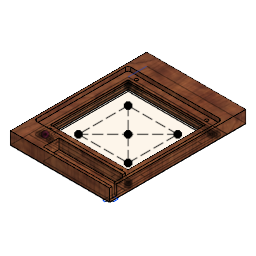
unicorn-frame-v34 (Autodesk Fusion 360 design; units mm, degrees)
Autodesk Fusion 360 part; units mm, degrees
sketch "Sketch1" plane through (0, 0, 0) normal (0, 0, 1) x (1, 0, 0)
  line L0 (0, 0) -> (254, 0)
  line L1 (254, 0) -> (254, 254)
  line L2 (254, 254) -> (0, 254)
  line L3 (0, 254) -> (0, 0)
  line L4 (279.4, 279.4) -> (-25.4, 279.4)
  line L5 (-25.4, 279.4) -> (-25.4, -25.4)
  line L6 (-25.4, -25.4) -> (279.4, -25.4)
  line L7 (279.4, -25.4) -> (279.4, 279.4)
  line L8 (246.0625, 246.0625) -> (7.9375, 246.0625)
  line L9 (7.9375, 246.0625) -> (7.9375, 7.9375)
  line L10 (7.9375, 7.9375) -> (246.0625, 7.9375)
  line L11 (246.0625, 7.9375) -> (246.0625, 246.0625)
  line L12 (258.7625, 265.1125) -> (-4.7625, 265.1125)
  line L13 (-11.1125, 258.7625) -> (-11.1125, -4.7625)
  line L14 (-4.7625, -11.1125) -> (258.7625, -11.1125)
  line L15 (265.1125, -4.7625) -> (265.1125, 258.7625)
  line L16 (39.6875, 0) -> (39.6875, -11.1125)
  line L17 (0, 39.6875) -> (-11.1125, 39.6875)
  line L18 (214.3125, 0) -> (214.3125, -11.1125)
  line L19 (254, 39.6875) -> (265.1125, 39.6875)
  line L20 (254, 214.3125) -> (265.1125, 214.3125)
  line L21 (214.3125, 254) -> (214.3125, 265.1125)
  line L22 (39.6875, 265.1125) -> (39.6875, 254)
  line L23 (-11.1125, 214.3125) -> (0, 214.3125)
  line L24 (263.525, 271.4625) -> (-9.525, 271.4625)
  line L25 (-17.4625, 263.525) -> (-17.4625, -9.525)
  line L26 (-9.525, -17.4625) -> (263.525, -17.4625)
  line L27 (271.4625, -9.525) -> (271.4625, 263.525)
  circle A0 centre (0, 0) radius 3.9688
  circle A1 centre (254, 0) radius 3.9688
  circle A2 centre (254, 254) radius 3.9688
  circle A3 centre (0, 254) radius 3.9688
  line L28 (0, 0) -> (0, -11.1125) construction
  line L29 (39.6875, -5.5563) -> (0, -5.5563) construction
  circle A4 centre (19.8437, -5.5563) radius 1.7145
  circle A5 centre (235.7437, -5.5563) radius 1.7145
  circle A6 centre (19.8437, 259.5562) radius 1.7145
  circle A7 centre (235.7437, 259.5562) radius 1.7145
  arc A8 (-11.1125, -4.7625) -> (-4.7625, -11.1125) centre (-4.7625, -4.7625) ccw
  arc A9 (258.7625, -11.1125) -> (265.1125, -4.7625) centre (258.7625, -4.7625) ccw
  arc A10 (265.1125, 258.7625) -> (258.7625, 265.1125) centre (258.7625, 258.7625) ccw
  arc A11 (-4.7625, 265.1125) -> (-11.1125, 258.7625) centre (-4.7625, 258.7625) ccw
  arc A12 (263.525, -17.4625) -> (271.4625, -9.525) centre (263.525, -9.525) ccw
  arc A13 (-17.4625, -9.525) -> (-9.525, -17.4625) centre (-9.525, -9.525) ccw
  arc A14 (-9.525, 271.4625) -> (-17.4625, 263.525) centre (-9.525, 263.525) ccw
  arc A15 (271.4625, 263.525) -> (263.525, 271.4625) centre (263.525, 263.525) ccw
  line L30 (263.525, -17.4625) -> (263.525, -25.4)
  line L31 (271.4625, -25.4) -> (271.4625, -9.525)
  line L32 (271.4625, -25.4) -> (271.4625, -87.515)
  line L33 (271.4625, -87.515) -> (263.525, -87.515)
  line L34 (263.525, -87.515) -> (263.525, -25.4)
  line L35 (203.2, 203.2) -> (50.8, 203.2) construction
  line L36 (50.8, 203.2) -> (50.8, 50.8) construction
  line L37 (50.8, 50.8) -> (203.2, 50.8) construction
  line L38 (203.2, 50.8) -> (203.2, 203.2) construction
  line L39 (203.2, 203.2) -> (50.8, 50.8) construction
  line L40 (50.8, 203.2) -> (203.2, 50.8) construction
  circle A16 centre (50.8, 203.2) radius 3.302
  circle A17 centre (203.2, 203.2) radius 3.302
  circle A18 centre (203.2, 50.8) radius 3.302
  circle A19 centre (50.8, 50.8) radius 3.302
  line L41 (241.3, 241.3) -> (12.7, 241.3)
  line L42 (12.7, 241.3) -> (12.7, 12.7)
  line L43 (12.7, 12.7) -> (241.3, 12.7)
  line L44 (241.3, 12.7) -> (241.3, 241.3)
  line L45 (279.4, -25.4) -> (279.4, -82.55)
  line L46 (279.4, -82.55) -> (-25.4, -82.55)
  line L47 (-25.4, -82.55) -> (-25.4, -25.4)
  line L48 (68.2625, -26.3525) -> (271.4625, -26.3525)
  line L49 (271.4625, -26.3525) -> (271.4625, -74.6125)
  line L50 (271.4625, -74.6125) -> (68.2625, -74.6125)
  line L51 (68.2625, -74.6125) -> (68.2625, -26.3525)
  line L52 (279.4, 279.4) -> (-25.4, 279.4)
  line L53 (-25.4, 279.4) -> (-25.4, 336.55)
  line L54 (-25.4, 336.55) -> (279.4, 336.55)
  line L55 (279.4, 336.55) -> (279.4, 279.4)
  line L56 (271.4625, -60.2191) -> (283.6575, -60.2191)
  line L57 (283.6575, -60.2191) -> (283.6575, -74.6125)
  line L58 (283.6575, -74.6125) -> (271.4625, -74.6125)
  line L59 (271.4625, -74.6125) -> (271.4625, -60.2191)
  dimension "d1" = 254
  dimension "d2" = 254
  dimension "d16" = 25.4
  dimension "d23" = 7.9375
  dimension "d30" = 50.8
  dimension "d31" = 50.8
  dimension "d32" = 50.8
  dimension "d33" = 50.8
  dimension "d34" = 50.8
  dimension "d35" = 50.8
  dimension "d36" = 50.8
  dimension "d37" = 50.8
  dimension "d51" = 7.9375
  dimension "d52" = 7.9375
  dimension "d53" = 7.9375
  dimension "d54" = 7.9375
  dimension "d55" = 3.429
  dimension "d58" = 215.9
  dimension "d59" = 265.1125
  dimension "d62" = 6.35
  dimension "d63" = 381
  dimension "d65" = 19.05
  dimension "d66" = 19.05
  dimension "d67" = 19.05
  dimension "d68" = 19.05
  dimension "d71" = 304.8
  dimension "d73" = 7.9375
  dimension "d75" = 7.9375
  dimension "d76" = 7.9375
  dimension "d77" = 7.9375
  dimension "d78" = 7.9375
  dimension "d79" = 7.9375
  dimension "d83" = 14.2875
  dimension "d86" = 127
  dimension "d87" = 127
  dimension "d88" = 152.4
  dimension "d89" = 152.4
  dimension "d90" = 6.604
  dimension "d91" = 6.604
  dimension "d92" = 6.604
  dimension "d93" = 6.604
  dimension "d94" = 12.7
  dimension "d95" = 57.15
  dimension "d103" = 48.26
  dimension "d104" = 203.2
  dimension "d107" = 7.9375
  dimension "d116" = 57.15
  measures "d30" distance of L14 L17
  measures "d31" distance of L13 L16
  measures "d32" distance of L12 L23
  measures "d33" distance of L13 L22
  measures "d34" distance of L15 L21
  measures "d35" distance of L12 L20
  measures "d36" distance of L14 L19
  measures "d37" distance of L15 L18
  measures "d51" diameter of A0
  measures "d52" diameter of A1
  measures "d53" diameter of A2
  measures "d54" diameter of A3
  measures "d55" diameter of A4
  measures "d62" radius of A8
  measures "d63" distance of L5 L7
  measures "d65" distance of L10 L14
  measures "d66" distance of L9 L13
  measures "d67" distance of L11 L15
  measures "d68" distance of L8 L12
  measures "d73" radius of A12
  measures "d75" distance of L7 L27
  measures "d76" distance of L6 L26
  measures "d77" distance of L5 L25
  measures "d78" distance of L4 L24
  measures "d79" distance of L30 L31
  measures "d83" distance of L14 L26
  measures "d90" diameter of A16
  measures "d91" diameter of A19
  measures "d92" diameter of A18
  measures "d93" diameter of A17
  measures "d95" distance of L6 L46
  measures "d103" distance of L48 L50
  measures "d104" distance of L49 L51
  measures "d107" distance of L46 L50
  measures "d116" distance of L52 L54
extrude "Extrude3" add sketch "Sketch1" along normal blind 6.35 contours L0 L3 A0 | L0 L3 A0 | L0 L1 L2 L3 A0 A1 A2 A3 | L0 L3 L13 L14 L16 L17 A0 A8 | L0 L14 L16 L18 | L3 L13 L17 L23 | L0 L1 L14 L15 L18 L19 A1 A9 | L2 L3 L12 L13 L22 L23 A3 A11 | L0 L1 A1 | L0 L1 A1 | L2 L3 A3 | L2 L3 A3 | L1 L15 L19 L20 | L2 L12 L21 L22 | L1 L2 L12 L15 L20 L21 A2 A10 | L1 L2 A2 | L1 L2 A2 | L4 L5 L6 L7 L24 L25 L26 L27 A13 A14 A15 L30 L31 L52 | L6 A12 L30 L31 | L24 L25 L26 L27 A12 A13 A14 A15 | A4 | A5 | A6 | A7 makes body 1
extrude "Extrude4" add sketch "Sketch1" along normal blind 12.7 from surface at 6.35 separate body contours L0 L3 A0 | L0 L1 L2 L3 A0 A1 A2 A3 | L0 L1 A1 | L2 L3 A3 | L1 L2 A2 | L8 L9 L10 L11 | A16 | A17 | A18 | A19 | L41 L42 L43 L44 picked at (2.1127, 1.5815) picked at (252.7352, 2.3163) picked at (1.2648, 251.6837) picked at (251.3676, 253.8117) makes body 2
extrude "Extrude5" add sketch "Sketch1" along normal blind 12.7 from surface at 6.35 separate body contours L0 L3 L13 L14 L16 L17 A0 A8 | L0 L1 L14 L15 L18 L19 A1 A9 | L2 L3 L12 L13 L22 L23 A3 A11 | L1 L2 L12 L15 L20 L21 A2 A10 makes body 3 at (258.0882, 226.2757, 19.05) makes body 4 at (-4.0882, 27.7243, 6.35) makes body 5 at (258.0882, 27.7243, 6.35) makes body 6 at (-4.0882, 226.2757, 6.35)
combine "Combine1" operation add target body 6 tool bodies 4 5 3 1
extrude "Extrude6" add sketch "Sketch1" along normal blind 25.4 contours L4 L5 L6 L7 L24 L25 L26 L27 A13 A14 A15 L30 L31 L52 bodies 6
extrude "Extrude7" add sketch "Sketch1" along normal blind 6.35 from surface at 19.05 separate body contours L0 L3 A0 | L0 L3 A0 | L0 L1 L2 L3 A0 A1 A2 A3 | L0 L3 L13 L14 L16 L17 A0 A8 | L0 L14 L16 L18 | L3 L13 L17 L23 | L0 L1 L14 L15 L18 L19 A1 A9 | L2 L3 L12 L13 L22 L23 A3 A11 | L0 L1 A1 | L0 L1 A1 | L2 L3 A3 | L2 L3 A3 | L1 L15 L19 L20 | L2 L12 L21 L22 | L1 L2 L12 L15 L20 L21 A2 A10 | L1 L2 A2 | L1 L2 A2 | L24 L25 L26 L27 A12 A13 A14 A15 | A4 | A5 | A6 | A7 makes body 7
extrude "Extrude8" add sketch "Sketch1" along normal blind 31.75 from surface at 6.35 contours L4 L5 L6 L7 L24 L25 L26 L27 A13 A14 A15 L30 L31 L52 bodies 6
extrude "Extrude9" cut sketch "Sketch1" along normal through all contours A4 | A5 | A6 | A7 bodies 7
chamfer "Chamfer1" distance 3.175 angle 45 4 edges at (234.1453, -4.9363, 25.4) (18.2453, -4.9363, 25.4) (234.1453, 260.1762, 25.4) (18.2453, 260.1762, 25.4) on bodies 7
extrude "Extrude16" add sketch "Sketch1" along normal blind 38.1 contours L4 L52 L53 L54 L55 | L6 L32 L45 L49 L56 | L6 L34 L46 L47 L48 L50 L51 | L6 L32 L34 L48 | L32 L45 L49 L56 L58 L59 | L32 L34 L48 L49 L50 L59 | L32 L45 L46 L58 | L34 L48 L50 L51 | L32 L34 L46 L50 bodies 6
extrude "Extrude17" cut sketch "Sketch1" along normal blind 31.75 from surface at 6.35 contours L6 L32 L34 L48 | L6 A12 L30 L31 | L32 L45 L49 L56 L58 L59 | L32 L34 L48 L49 L50 L59 | L34 L48 L50 L51 bodies 6
equation "d1 = d2"
equation "d16 = d66 + 1/4\""
equation "d23 = 5/16\""
equation "d24 = 1/4\""
equation "d26 = 1/4\""
equation "d27 = 1/2\""
equation "d29 = 5/8\""
equation "d31 = d30"
equation "d32 = d30"
equation "d33 = d30"
equation "d34 = d30"
equation "d35 = d30"
equation "d36 = d30"
equation "d37 = d30"
equation "d38 = 1/4\""
equation "d39 = 1/2\""
equation "d41 = d29 + 3/8\""
equation "d44 = 3/4\""
equation "d45 = 1/4\""
equation "d48 = 1/4\""
equation "d51 = 5/16\""
equation "d52 = d51"
equation "d53 = d51"
equation "d54 = d51"
equation "d58 = d2 - 1.5 in"
equation "d59 = d2 + 7/16\""
equation "d61 = 1/8\""
equation "d62 = 1/4\""
equation "d63 = 15\""
equation "d65 = d66"
equation "d66 = 3/4\""
equation "d67 = d65"
equation "d68 = d66"
equation "d71 = 12\""
equation "d73 = 5/16\""
equation "d75 = 5/16\""
equation "d76 = d75"
equation "d77 = d75"
equation "d78 = d75"
equation "d79 = 5/16\""
equation "d83 = 9/16\""
equation "d84 = 6 1/16\""
equation "d86 = d2 / 2"
equation "d87 = d86"
equation "d89 = d88"
equation "d91 = d90"
equation "d92 = d90"
equation "d93 = d90"
equation "d107 = 5/16\""
equation "d116 = d95"
equation "d117 = 1 1/2\""
equation "d119 = 1/4\""
equation "d120 = 1 1/4\""
named bodies: "sheets", "main", "backer"
